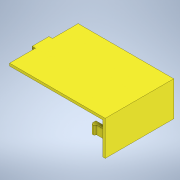
# Autodesk Inventor part: top
Saved by Autodesk Inventor 2022.2 (Build 262287000, 287)
## iProperties
Created: 2021-12-01
Part Number: top
Material: Generic
Document SubType Name: Modeling
Designer: samlo
Density: 1 g/cm^3
Appearance: Canary
Author: samlo
Autodesk Inventor part; units mm, degrees
ref_plane "YZ Plane" through (0, 0, 0) normal (1, 0, 0) x (0, 1, 0)
ref_plane "XZ Plane" through (0, 0, 0) normal (0, 1, 0) x (-1, 0, 0)
ref_plane "XY Plane" through (0, 0, 0) normal (0, 0, 1) x (1, 0, 0)
sketch "Sketch5" plane through (0, 0, 0) normal (0, 0, 1) x (1, 0, 0)
  line L0 (0, 0) -> (3, 0)
  line L1 (3, 0) -> (3, 41)
  line L2 (3, 41) -> (-110, 41)
  line L3 (-110, 41) -> (-110, 38)
  line L4 (-110, 38) -> (0, 38)
  line L5 (0, 38) -> (0, 0)
  dimension "d32" = 3
  dimension "d33" = 3
  dimension "d34" = 110
  dimension "d35" = 41
  constraints: 12 end point, 4 perpendicular, 1 horizontal
  measures "d32" distance of L0.start L0.end
  measures "d33" distance of L2.end L3.end
  measures "d34" distance of L3.end L4.end
  measures "d35" distance of L0.end L1.end
extrude "Extrusion4" add sketch "Sketch5" along normal blind 81
sketch "Sketch6" plane through (-110, 38, 0) normal (-1, 0, 0) x (0, 0, 1)
  line L0 (0, 0) -> (81, 0) projected
  line L1 (0, 3) -> (81, 3) projected
  line L2 (30.5, 0) -> (50.5, 0)
  line L3 (50.5, 0) -> (50.5, 3)
  line L4 (50.5, 3) -> (30.5, 3)
  line L5 (30.5, 3) -> (30.5, 0)
  point P0 (0, -38)
  point P1 (30.5, 3)
  dimension "d38" = 20
  dimension "d39" = 30.5
  constraints: 8 end point, 2 parallel, 2 point on line, 1 horizontal, 1 perpendicular
  measures "d38" distance of L2.start L2.end
  measures "d39" distance of L0.end L2.end
extrude "Extrusion5" add sketch "Sketch6" along normal blind 4
sketch "Sketch11" plane through (0, 0, 0) normal (-1, 0, 0) x (0, 0, 1)
  line L0 (81, 0) -> (81, 41) projected
  line L1 (78, 26) -> (74, 26)
  line L2 (74, 26) -> (74, 16)
  line L3 (74, 16) -> (77, 16)
  line L4 (0, 0) -> (81, 0) projected
  line L5 (78, 26) -> (78, 16)
  line L6 (81, 38) -> (81, 0) projected
  line L7 (78, 16) -> (77, 16)
  point P0 (81, 26)
  point P1 (81, 16)
  dimension "d82" = 4
  dimension "d83" = 10
  dimension "d84" = 16
  dimension "d85" = 74
  constraints: 10 end point, 2 parallel, 1 collinear, 1 horizontal, 1 perpendicular, 1 point on line
  measures "d82" distance of L1.start L1.end
  measures "d83" distance of L2.end L1.end
  measures "d84" distance from line of L3.end L4
  measures "d85" horizontal distance of L2.end L4.start
extrude "Extrusion6" add sketch "Sketch11" along normal blind 15
ref_plane "Work Plane3" through (0, 0, 40.5) normal (0, 0, 1) x (1, 0, 0)
mirror "Mirror4" about plane through (0, 0, 40.5) normal (0, 0, 1) of "Extrusion6"
sketch "Sketch15" plane through (0, 16, 74) normal (0, -1, 0) x (1, 0, 0)
  line L0 (0, 4) -> (-15, 4) projected
  line L1 (-15, 4) -> (-13.3218, 6)
  line L2 (-13.3218, 6) -> (-11.6782, 6)
  line L3 (-11.6782, 6) -> (-10, 4)
  line L4 (-15, 0) -> (-15, 4) projected
  line L5 (-15, 4) -> (-10, 4)
  line L6 (0, -74) -> (0, 7) projected
  dimension "d86" = 10
  dimension "d87" = 50
  dimension "d88" = 50
  dimension "d89" = 2
  constraints: 8 end point, 1 parallel, 1 perpendicular, 1 point on line
  measures "d86" distance from line of L6 L3.end
  measures "d87" angle of L0 L1
  measures "d88" angle of L0 L3
  measures "d89" distance between parallel lines of L0 L2
extrude "Extrusion10" add sketch "Sketch15" against normal up to surface (10 mm away)
mirror "Mirror8" about plane through (0, 0, 40.5) normal (0, 0, 1) of "Extrusion10"
body "Solid2"
